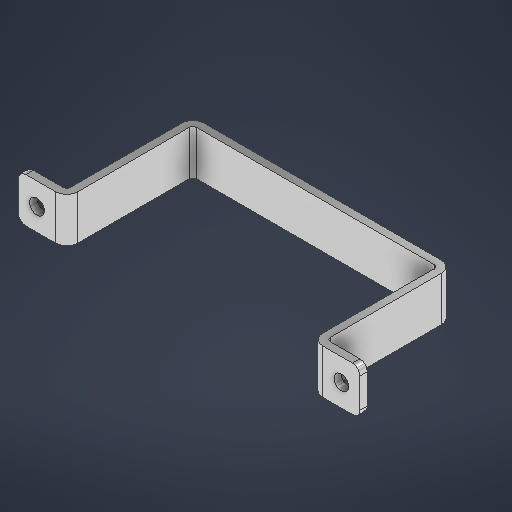
# Autodesk Inventor part: Handle
Saved by Autodesk Inventor 2026.1 (Build 301233000, 233)
## iProperties
Created: 2025-12-10
Part Number: Handle
Material: Generisch
Document SubType Name: Modeling
Designer: Familie
Density: 1 g/cm^3
Appearance: Chrom - poliert
Author: Familie
Autodesk Inventor part; units mm, degrees
ref_plane "YZ Plane" through (0, 0, 0) normal (1, 0, 0) x (0, 1, 0)
ref_plane "XZ Plane" through (0, 0, 0) normal (0, 1, 0) x (-1, 0, 0)
sketch "Skizze1" plane through (0, 0, 0) normal (0, 0, 1) x (1, 0, 0)
  line L0 (12, 2) -> (12, 32)
  line L1 (80, 2) -> (80, 32)
  arc A0 (14, 34) -> (12, 32) centre (14, 32) ccw
  arc A1 (80, 32) -> (78, 34) centre (78, 32) ccw
  line L2 (10, 0) -> (0, 0)
  line L3 (82, 0) -> (92, 0)
  arc A2 (80, 2) -> (82, 0) centre (82, 2) ccw
  arc A3 (10, 0) -> (12, 2) centre (10, 2) ccw
  line L4 (78, 34) -> (14, 34)
  dimension "d1" = 30
  dimension "d2" = 30
  dimension "d3" = 2
  dimension "d7" = 2
  dimension "d29" = 2
  dimension "d30" = 2
  dimension "d31" = 92
  dimension "d32" = 10
  dimension "d33" = 10
  constraints: 10 end point, 8 point on circle, 8 tangent, 4 centre point, 4 horizontal, 1 parallel, 1 vertical
  measures "d1" distance of L0.start L0.end
  measures "d2" distance of L1.start L1.end
  measures "d3" horizontal distance of L4.end L0.end
  measures "d7" horizontal distance of L4.start L1.end
  measures "d29" distance from line of L3.start L1
  measures "d30" distance from line of L2.start L0
  measures "d31" distance of L3.end L2.end
  measures "d32" distance of L3.start L3.end
  measures "d33" distance of L2.end L2.start
ref_plane "Arbeitsebene1" through (0, 0, 0) normal (-1, 0, 0) x (0, -1, 0)
sketch "Skizze2" plane through (0, 0, 0) normal (-1, 0, 0) x (0, -1, 0)
  line L0 (-1, 6) -> (1, 6)
  line L1 (1, 6) -> (1, -6)
  line L2 (1, -6) -> (-1, -6)
  line L3 (-1, -6) -> (-1, 6)
  point P0 (0, 0)
  point P1 (1, 0)
  dimension "d15" = 12
  dimension "d16" = 6
  dimension "d17" = 1
  dimension "d18" = 2
  constraints: 8 end point, 2 parallel, 1 horizontal, 1 midpoint, 1 perpendicular
  measures "d15" distance of L0.end L1.end
  measures "d16" distance from line of point (0, 0) L2
  measures "d17" distance from line of point (0, 0) L1
  measures "d18" distance from line of point (1, 0) L3
sweep "Sweeping1" add profiles "Skizze2" path "Skizze1"
sketch "Skizze4" plane through (0, -1, 6) normal (0, -1, 0) x (1, 0, 0)
  circle A0 centre (5, -6) radius 2
  circle A1 centre (87, -6) radius 2
  line L0 (0, -12) -> (0, 0) projected
  line L1 (92, -12) -> (92, 0) projected
  line L2 (92, 0) -> (82, 0) projected
  point P0 (0, -6)
  dimension "d37" = 4
  dimension "d38" = 4
  dimension "d39" = 5
  dimension "d40" = 5
  dimension "d41" = 6
  constraints: 2 centre point, 1 horizontal alignment
  measures "d37" diameter of A0
  measures "d38" diameter of A1
  measures "d39" distance from line of L0 A0.centre
  measures "d40" distance from line of A1.centre L1
  measures "d41" distance from line of L2 A1.centre
extrude "Extrusion2" cut sketch "Skizze4" against normal blind 4
fillet "Rundung1" radius 2 4 edges at (92, 0, -6) (92, 0, 6) (0, 0, -6) (0, 0, 6)
equation "\"d1\" = d2"
equation "\"d3\" = d4"
equation "\"d7\" = d4"
equation "\"d4\" = 2"
